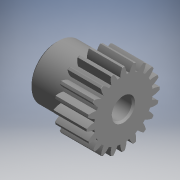
# Autodesk Inventor part: PS1-20_On
Saved by Autodesk Inventor 2017.3 (Build 213256000, 256)
## iProperties
Part Number: PS1-20_On
Material: Generic
Catalog Web Link: www.cadenas.de
Description: Plastic Spur Gears (PS)-
Vendor: KHK
Document SubType Name: Modeling
Designer: partserver
Manufacturer: KHK
Mass: 4.50562 g
Surface Area: 26.5724 cm^2
Volume: 4.50562 cm^3
Density: 1 g/cm^3
Appearance: PSOLRGB-175-175-175
Category: PARTsolutions
Company: KHK
Title: PS1-20
Author: Cadenas PARTsolutions
PSOL_IDENT_0: {$CADENAS_DATA\23d-libs\khk\spur_gears\plastic_spur_gears_ps.prj},177 {VTYP=3D},{NB=PS1-20_On},{LINA=
PSOL_IDENT_1: PS1-20},{NN=Plastic Spur Gears (PS)},{DATE=10.04.2020 06:07:24},{GEOMDATE=05.07.2019 08:26:52},{VERS
PSOL_IDENT_2: ION=},{LINEID=50},{WBVAR=TOOTH},{WBNUMERIC=}  {NB=PS1-20_On},{LINA=PS1-20},{KT=DUMMY},{CN=PS1-20},{M=
PSOL_IDENT_3: 1},{MX=1.000},{Z=20},{S=S1},{A=6},{B=16},{C=20.0},{D=22.0},{E=10},{F=10},{G=20},{K=0},{KD=0.0},{M1=0
PSOL_IDENT_4: },{SCSX=0},{J=0.0},{WMF=S1003.WMF},{R=0.6},{N=0.5},{L=0.1},{L2=0.5},{CBD1=0.0},{CBD2=0.0},{TOOTH=On}
NB: PS1-20_On
NN: Plastic Spur Gears (PS)
NBSYN: $CN._$TOOTH.
LINA: PS1-20
CATALOG: KHK
CN: PS1-20
M: 1
Z: 20
S: S1
A: 6
B: 16
C: 20
D: 22
E: 10
F: 10
G: 20
K: 0
KD: 0
M1: 0
J: 0
TOOTH: On
SUPPLIER: KHK
ARTICLENO: PS1-20_On
BOMINFO: PS1-20
CREATOR: CADENAS GmbH
Autodesk Inventor part; units mm, degrees
ref_plane "YZ Plane" through (0, 0, 0) normal (1, 0, 0) x (0, 1, 0)
ref_plane "XZ Plane" through (0, 0, 0) normal (0, 1, 0) x (-1, 0, 0)
ref_plane "XY Plane" through (0, 0, 0) normal (0, 0, 1) x (1, 0, 0)
sketch "Sketch_8" plane through (0, 0, 0) normal (0, 0, 1) x (1, 0, 0)
  line L0 (20, 0) -> (0, 0)
  line L1 (0, 3.5) -> (0.5, 3)
  line L2 (0.5, 3) -> (19.5, 3)
  line L3 (19.5, 3) -> (20, 3.5)
  line L4 (20, 3.5) -> (20, 7.5)
  line L5 (20, 7.5) -> (19.5, 8)
  line L6 (19.5, 8) -> (10.6, 8)
  arc A0 (10, 8.6) -> (10.6, 8) centre (10.6, 8.6) ccw
  line L7 (10, 8.6) -> (10, 10.9)
  line L8 (10, 10.9) -> (9.9, 11)
  line L9 (9.9, 11) -> (0.1, 11)
  line L10 (0.1, 11) -> (0, 10.9)
  line L11 (0, 10.9) -> (0, 3.5)
  constraints: 24 end point, 2 point on circle, 1 centre point
revolve "Revolution1" add sketch "Sketch_8" angle 360 about axis through (20, 0, 0) along (1, 0, 0)
sketch "Sketch_11" plane through (0, 0, 0) normal (1, 0, 0) x (0, 1, 0)
  line L0 (22, 22) -> (-22, 22)
  line L1 (-22, 22) -> (-22, -22)
  line L2 (-22, -22) -> (22, -22)
  line L3 (22, -22) -> (22, 22)
  arc A0 (0.3455, 10.9946) -> (-0.3455, 10.9946) centre (0, 0) ccw
  arc A1 (-0.3455, 10.9946) -> (-0.9602, 8.6972) centre (5.0283, 8.3259) ccw
  arc A2 (-0.9602, 8.6972) -> (-1.7744, 8.5682) centre (0, 0) ccw
  arc A3 (-1.7744, 8.5682) -> (-3.0689, 10.5632) centre (-7.3551, 6.3646) ccw
  arc A4 (-3.0689, 10.5632) -> (-3.7261, 10.3497) centre (0, 0) ccw
  arc A5 (-3.7261, 10.3497) -> (-3.6008, 7.9748) centre (2.2094, 9.4722) ccw
  arc A6 (-3.6008, 7.9748) -> (-4.3353, 7.6005) centre (0, 0) ccw
  arc A7 (-4.3353, 7.6005) -> (-6.1829, 9.0979) centre (-8.9618, 3.7802) ccw
  arc A8 (-6.1829, 9.0979) -> (-6.742, 8.6917) centre (0, 0) ccw
  arc A9 (-6.742, 8.6917) -> (-5.8889, 6.4718) centre (-0.8258, 9.6914) ccw
  arc A10 (-5.8889, 6.4718) -> (-6.4718, 5.8889) centre (0, 0) ccw
  arc A11 (-6.4718, 5.8889) -> (-8.6917, 6.742) centre (-9.6914, 0.8258) ccw
  arc A12 (-8.6917, 6.742) -> (-9.0979, 6.1829) centre (0, 0) ccw
  arc A13 (-9.0979, 6.1829) -> (-7.6005, 4.3353) centre (-3.7802, 8.9618) ccw
  arc A14 (-7.6005, 4.3353) -> (-7.9748, 3.6008) centre (0, 0) ccw
  arc A15 (-7.9748, 3.6008) -> (-10.3497, 3.7261) centre (-9.4722, -2.2094) ccw
  arc A16 (-10.3497, 3.7261) -> (-10.5632, 3.0689) centre (0, 0) ccw
  arc A17 (-10.5632, 3.0689) -> (-8.5682, 1.7744) centre (-6.3646, 7.3551) ccw
  arc A18 (-8.5682, 1.7744) -> (-8.6972, 0.9602) centre (0, 0) ccw
  arc A19 (-8.6972, 0.9602) -> (-10.9946, 0.3455) centre (-8.3259, -5.0283) ccw
  arc A20 (-10.9946, 0.3455) -> (-10.9946, -0.3455) centre (0, 0) ccw
  arc A21 (-10.9946, -0.3455) -> (-8.6972, -0.9602) centre (-8.3259, 5.0283) ccw
  arc A22 (-8.6972, -0.9602) -> (-8.5682, -1.7744) centre (0, 0) ccw
  arc A23 (-8.5682, -1.7744) -> (-10.5632, -3.0689) centre (-6.3646, -7.3551) ccw
  arc A24 (-10.5632, -3.0689) -> (-10.3497, -3.7261) centre (0, 0) ccw
  arc A25 (-10.3497, -3.7261) -> (-7.9748, -3.6008) centre (-9.4722, 2.2094) ccw
  arc A26 (-7.9748, -3.6008) -> (-7.6005, -4.3353) centre (0, 0) ccw
  arc A27 (-7.6005, -4.3353) -> (-9.0979, -6.1829) centre (-3.7802, -8.9618) ccw
  arc A28 (-9.0979, -6.1829) -> (-8.6917, -6.742) centre (0, 0) ccw
  arc A29 (-8.6917, -6.742) -> (-6.4718, -5.8889) centre (-9.6914, -0.8258) ccw
  arc A30 (-6.4718, -5.8889) -> (-5.8889, -6.4718) centre (0, 0) ccw
  arc A31 (-5.8889, -6.4718) -> (-6.742, -8.6917) centre (-0.8258, -9.6914) ccw
  arc A32 (-6.742, -8.6917) -> (-6.1829, -9.0979) centre (0, 0) ccw
  arc A33 (-6.1829, -9.0979) -> (-4.3353, -7.6005) centre (-8.9618, -3.7802) ccw
  arc A34 (-4.3353, -7.6005) -> (-3.6008, -7.9748) centre (0, 0) ccw
  arc A35 (-3.6008, -7.9748) -> (-3.7261, -10.3497) centre (2.2094, -9.4722) ccw
  arc A36 (-3.7261, -10.3497) -> (-3.0689, -10.5632) centre (0, 0) ccw
  arc A37 (-3.0689, -10.5632) -> (-1.7744, -8.5682) centre (-7.3551, -6.3646) ccw
  arc A38 (-1.7744, -8.5682) -> (-0.9602, -8.6972) centre (0, 0) ccw
  arc A39 (-0.9602, -8.6972) -> (-0.3455, -10.9946) centre (5.0283, -8.3259) ccw
  arc A40 (-0.3455, -10.9946) -> (0.3455, -10.9946) centre (0, 0) ccw
  arc A41 (0.3455, -10.9946) -> (0.9602, -8.6972) centre (-5.0283, -8.3259) ccw
  arc A42 (0.9602, -8.6972) -> (1.7744, -8.5682) centre (0, 0) ccw
  arc A43 (1.7744, -8.5682) -> (3.0689, -10.5632) centre (7.3551, -6.3646) ccw
  arc A44 (3.0689, -10.5632) -> (3.7261, -10.3497) centre (0, 0) ccw
  arc A45 (3.7261, -10.3497) -> (3.6008, -7.9748) centre (-2.2094, -9.4722) ccw
  arc A46 (3.6008, -7.9748) -> (4.3353, -7.6005) centre (0, 0) ccw
  arc A47 (4.3353, -7.6005) -> (6.1829, -9.0979) centre (8.9618, -3.7802) ccw
  arc A48 (6.1829, -9.0979) -> (6.742, -8.6917) centre (0, 0) ccw
  arc A49 (6.742, -8.6917) -> (5.8889, -6.4718) centre (0.8258, -9.6914) ccw
  arc A50 (5.8889, -6.4718) -> (6.4718, -5.8889) centre (0, 0) ccw
  arc A51 (6.4718, -5.8889) -> (8.6917, -6.742) centre (9.6914, -0.8258) ccw
  arc A52 (8.6917, -6.742) -> (9.0979, -6.1829) centre (0, 0) ccw
  arc A53 (9.0979, -6.1829) -> (7.6005, -4.3353) centre (3.7802, -8.9618) ccw
  arc A54 (7.6005, -4.3353) -> (7.9748, -3.6008) centre (0, 0) ccw
  arc A55 (7.9748, -3.6008) -> (10.3497, -3.7261) centre (9.4722, 2.2094) ccw
  arc A56 (10.3497, -3.7261) -> (10.5632, -3.0689) centre (0, 0) ccw
  arc A57 (10.5632, -3.0689) -> (8.5682, -1.7744) centre (6.3646, -7.3551) ccw
  arc A58 (8.5682, -1.7744) -> (8.6972, -0.9602) centre (0, 0) ccw
  arc A59 (8.6972, -0.9602) -> (10.9946, -0.3455) centre (8.3259, 5.0283) ccw
  arc A60 (10.9946, -0.3455) -> (10.9946, 0.3455) centre (0, 0) ccw
  arc A61 (10.9946, 0.3455) -> (8.6972, 0.9602) centre (8.3259, -5.0283) ccw
  arc A62 (8.6972, 0.9602) -> (8.5682, 1.7744) centre (0, 0) ccw
  arc A63 (8.5682, 1.7744) -> (10.5632, 3.0689) centre (6.3646, 7.3551) ccw
  arc A64 (10.5632, 3.0689) -> (10.3497, 3.7261) centre (0, 0) ccw
  arc A65 (10.3497, 3.7261) -> (7.9748, 3.6008) centre (9.4722, -2.2094) ccw
  arc A66 (7.9748, 3.6008) -> (7.6005, 4.3353) centre (0, 0) ccw
  arc A67 (7.6005, 4.3353) -> (9.0979, 6.1829) centre (3.7802, 8.9618) ccw
  arc A68 (9.0979, 6.1829) -> (8.6917, 6.742) centre (0, 0) ccw
  arc A69 (8.6917, 6.742) -> (6.4718, 5.8889) centre (9.6914, 0.8258) ccw
  arc A70 (6.4718, 5.8889) -> (5.8889, 6.4718) centre (0, 0) ccw
  arc A71 (5.8889, 6.4718) -> (6.742, 8.6917) centre (0.8258, 9.6914) ccw
  arc A72 (6.742, 8.6917) -> (6.1829, 9.0979) centre (0, 0) ccw
  arc A73 (6.1829, 9.0979) -> (4.3353, 7.6005) centre (8.9618, 3.7802) ccw
  arc A74 (4.3353, 7.6005) -> (3.6008, 7.9748) centre (0, 0) ccw
  arc A75 (3.6008, 7.9748) -> (3.7261, 10.3497) centre (-2.2094, 9.4722) ccw
  arc A76 (3.7261, 10.3497) -> (3.0689, 10.5632) centre (0, 0) ccw
  arc A77 (3.0689, 10.5632) -> (1.7744, 8.5682) centre (7.3551, 6.3646) ccw
  arc A78 (1.7744, 8.5682) -> (0.9602, 8.6972) centre (0, 0) ccw
  arc A79 (0.9602, 8.6972) -> (0.3455, 10.9946) centre (-5.0283, 8.3259) ccw
  constraints: 160 point on circle, 80 centre point, 8 end point
extrude "Extrusion1" cut sketch "Sketch_11" along normal blind 10
body "Solid1"
